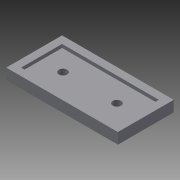
# Autodesk Inventor part: castor_bracket
Saved by Autodesk Inventor 2015 (Build 190159000, 159)
## iProperties
Created: 2014-11-12
Part Number: castor_bracket
Material: Generic
Document SubType Name: Modeling
Designer: Colin
Density: 1 g/cm^3
Appearance: Default
Author: Colin
Autodesk Inventor part; units mm, degrees
ref_plane "YZ Plane" through (0, 0, 0) normal (1, 0, 0) x (0, 1, 0)
ref_plane "XZ Plane" through (0, 0, 0) normal (0, 1, 0) x (-1, 0, 0)
ref_plane "XY Plane" through (0, 0, 0) normal (0, 0, 1) x (1, 0, 0)
sketch "Sketch1" plane through (0, 0, 0) normal (0, 1, 0) x (-1, 0, 0)
  line L0 (0, 0) -> (-30.48, 0)
  line L1 (-30.48, 0) -> (-30.48, -15.24)
  line L2 (-30.48, -15.24) -> (0, -15.24)
  line L3 (0, -15.24) -> (0, 0)
  line L4 (0, -7.62) -> (-30.48, -7.62) construction
  circle A0 centre (-7.874, -7.62) radius 1.143
  circle A1 centre (-22.606, -7.62) radius 1.143
  dimension "d0" = 15.24
  dimension "d1" = 30.48
  dimension "d2" = 2.286
  dimension "d3" = 2.286
  dimension "d4" = 14.732
  dimension "d5" = 7.874
  constraints: 10 end point, 2 centre point, 2 midpoint, 2 parallel, 2 point on line, 1 horizontal, 1 perpendicular
  measures "d0" distance of L2.end L0.start
  measures "d1" distance of L0.start L0.end
  measures "d2" diameter of A1
  measures "d3" diameter of A0
  measures "d4" distance of A1.centre A0.centre
  measures "d5" distance from line of L3 A0.centre
extrude "Extrusion1" add sketch "Sketch1" along normal blind 2.032
sketch "Sketch2" plane through (0, 2.032, 0) normal (0, 1, 0) x (1, 0, 0)
  line L0 (0, 0) -> (30.48, 0)
  line L1 (30.48, 0) -> (30.48, 15.24)
  line L2 (30.48, 15.24) -> (0, 15.24)
  line L3 (0, 15.24) -> (0, 0)
  line L4 (2.032, 2.032) -> (28.448, 2.032)
  line L5 (28.448, 2.032) -> (28.448, 13.208)
  line L6 (28.448, 13.208) -> (2.032, 13.208)
  line L7 (2.032, 13.208) -> (2.032, 2.032)
  dimension "d8" = 2.032
  dimension "d9" = 2.032
  dimension "d10" = 2.032
  dimension "d12" = 2.032
  constraints: 16 end point, 4 parallel, 2 horizontal, 2 perpendicular
  measures "d8" distance between parallel lines of L3 L7
  measures "d9" distance between parallel lines of L0 L4
  measures "d10" distance between parallel lines of L2 L6
  measures "d12" distance between parallel lines of L1 L5
extrude "Extrusion2" add sketch "Sketch2" along normal blind 0.9398
body "Solid1"
